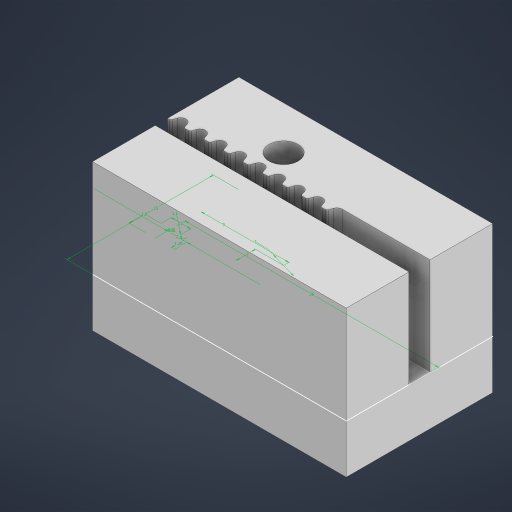
# Autodesk Inventor part: Y Axis Carriage
Saved by Autodesk Inventor 2024 (Build 280153000, 153)
## iProperties
Created: 2024-10-02
Part Number: Y Axis Carriage
Material: Generic
Document SubType Name: Modeling
Designer: jerem
Density: 1 g/cm^3
Appearance: Default
Author: jerem
Autodesk Inventor part; units mm, degrees
ref_plane "YZ Plane" through (0, 0, 0) normal (1, 0, 0) x (0, 1, 0)
ref_plane "XZ Plane" through (0, 0, 0) normal (0, 1, 0) x (-1, 0, 0)
ref_plane "XY Plane" through (0, 0, 0) normal (0, 0, 1) x (1, 0, 0)
sketch "Sketch1" plane through (0, 0, 0) normal (0, 1, 0) x (-1, 0, 0)
  line L0 (0, 0) -> (0, -1.075)
  line L1 (0, 0) -> (0, 1.075) construction
  line L2 (0, -1.075) -> (-26, -1.075) construction
  line L3 (0, 1.075) -> (-26, 1.075)
  line L4 (0, 1.075) -> (0, 7.5) construction
  line L5 (0, -1.075) -> (0, -7.5) construction
  line L6 (-26, -1.075) -> (-26, 1.075)
  line L7 (0, 1.075) -> (0, 7.5)
  line L8 (0, 7.5) -> (-26, 7.5)
  line L9 (-26, 7.5) -> (-26, 1.075)
  line L10 (0, -7.5) -> (-26, -7.5)
  line L11 (-26, -7.5) -> (-26, -1.075)
  line L12 (1, -0.525) -> (1, 1.075) construction
  arc A0 (-1.5221, -0.698) -> (-0.4779, -0.698) centre (-1, -0.525) ccw
  line L13 (0, -0.175) -> (-0.1602, -0.175)
  line L14 (-0.35, -0.3121) -> (-0.4779, -0.698)
  line L15 (-1, -0.525) -> (1, -0.525) construction
  line L16 (0, -0.525) -> (0, -0.175) construction
  arc A1 (-0.1602, -0.175) -> (-0.35, -0.3121) centre (-0.1602, -0.375) ccw
  line L17 (-1, -0.525) -> (-1, 0) construction
  line L18 (-1, -0.525) -> (-1, 0.025) construction
  line L19 (-2, -0.175) -> (-1.8398, -0.175)
  line L20 (-1.65, -0.3121) -> (-1.5221, -0.698)
  arc A2 (-1.65, -0.3121) -> (-1.8398, -0.175) centre (-1.8398, -0.375) ccw
  line L21 (-2, -0.175) -> (-2.1602, -0.175)
  arc A3 (-2.1602, -0.175) -> (-2.35, -0.3121) centre (-2.1602, -0.375) ccw
  line L22 (-2.35, -0.3121) -> (-2.4779, -0.698)
  arc A4 (-3.5221, -0.698) -> (-2.4779, -0.698) centre (-3, -0.525) ccw
  line L23 (-3.65, -0.3121) -> (-3.5221, -0.698)
  arc A5 (-3.65, -0.3121) -> (-3.8398, -0.175) centre (-3.8398, -0.375) ccw
  line L24 (-4, -0.175) -> (-3.8398, -0.175)
  line L25 (-4, -0.175) -> (-4.1602, -0.175)
  arc A6 (-4.1602, -0.175) -> (-4.35, -0.3121) centre (-4.1602, -0.375) ccw
  line L26 (-4.35, -0.3121) -> (-4.4779, -0.698)
  arc A7 (-5.5221, -0.698) -> (-4.4779, -0.698) centre (-5, -0.525) ccw
  line L27 (-5.65, -0.3121) -> (-5.5221, -0.698)
  arc A8 (-5.65, -0.3121) -> (-5.8398, -0.175) centre (-5.8398, -0.375) ccw
  line L28 (-6, -0.175) -> (-5.8398, -0.175)
  line L29 (-6, -0.175) -> (-6.1602, -0.175)
  arc A9 (-6.1602, -0.175) -> (-6.35, -0.3121) centre (-6.1602, -0.375) ccw
  line L30 (-6.35, -0.3121) -> (-6.4779, -0.698)
  arc A10 (-7.5221, -0.698) -> (-6.4779, -0.698) centre (-7, -0.525) ccw
  line L31 (-7.65, -0.3121) -> (-7.5221, -0.698)
  arc A11 (-7.65, -0.3121) -> (-7.8398, -0.175) centre (-7.8398, -0.375) ccw
  line L32 (-8, -0.175) -> (-7.8398, -0.175)
  line L33 (-8, -0.175) -> (-8.1602, -0.175)
  arc A12 (-8.1602, -0.175) -> (-8.35, -0.3121) centre (-8.1602, -0.375) ccw
  line L34 (-8.35, -0.3121) -> (-8.4779, -0.698)
  arc A13 (-9.5221, -0.698) -> (-8.4779, -0.698) centre (-9, -0.525) ccw
  line L35 (-9.65, -0.3121) -> (-9.5221, -0.698)
  arc A14 (-9.65, -0.3121) -> (-9.8398, -0.175) centre (-9.8398, -0.375) ccw
  line L36 (-10, -0.175) -> (-9.8398, -0.175)
  line L37 (-10, -0.175) -> (-10.1602, -0.175)
  arc A15 (-10.1602, -0.175) -> (-10.35, -0.3121) centre (-10.1602, -0.375) ccw
  line L38 (-10.35, -0.3121) -> (-10.4779, -0.698)
  arc A16 (-11.5221, -0.698) -> (-10.4779, -0.698) centre (-11, -0.525) ccw
  line L39 (-11.65, -0.3121) -> (-11.5221, -0.698)
  arc A17 (-11.65, -0.3121) -> (-11.8398, -0.175) centre (-11.8398, -0.375) ccw
  line L40 (-12, -0.175) -> (-11.8398, -0.175)
  line L41 (-12, -0.175) -> (-12.1602, -0.175)
  arc A18 (-12.1602, -0.175) -> (-12.35, -0.3121) centre (-12.1602, -0.375) ccw
  line L42 (-12.35, -0.3121) -> (-12.4779, -0.698)
  arc A19 (-13.5221, -0.698) -> (-12.4779, -0.698) centre (-13, -0.525) ccw
  line L43 (-13.65, -0.3121) -> (-13.5221, -0.698)
  arc A20 (-13.65, -0.3121) -> (-13.8398, -0.175) centre (-13.8398, -0.375) ccw
  line L44 (-14, -0.175) -> (-13.8398, -0.175)
  line L45 (-14, -0.175) -> (-14.1602, -0.175)
  arc A21 (-14.1602, -0.175) -> (-14.35, -0.3121) centre (-14.1602, -0.375) ccw
  line L46 (-14.35, -0.3121) -> (-14.4779, -0.698)
  arc A22 (-15.5221, -0.698) -> (-14.4779, -0.698) centre (-15, -0.525) ccw
  line L47 (-15.65, -0.3121) -> (-15.5221, -0.698)
  arc A23 (-15.65, -0.3121) -> (-15.8398, -0.175) centre (-15.8398, -0.375) ccw
  line L48 (-16, -0.175) -> (-15.8398, -0.175)
  line L49 (-16, -0.175) -> (-16, -1.075) construction
  circle A24 centre (-9, -3.075) radius 1.5
  line L50 (-16, -1.075) -> (-26, -1.075)
  line L51 (0, -1.075) -> (0, -7.5)
  line L52 (-9, -3.075) -> (-9, -1.075) construction
  arc A25 (-17, -1.075) -> (-16.4779, -0.698) centre (-17, -0.525) ccw
  line L53 (-16.35, -0.3121) -> (-16.4779, -0.698)
  arc A26 (-16.1602, -0.175) -> (-16.35, -0.3121) centre (-16.1602, -0.375) ccw
  line L54 (-16, -0.175) -> (-16.1602, -0.175)
  line L55 (0, 0) -> (0, 1.075)
  point P0 (0, -0.5375)
  point P1 (-0.3046, -0.175)
  point P2 (-2.3046, -0.175)
  point P3 (-4.3046, -0.175)
  point P4 (-6.3046, -0.175)
  point P5 (-8.3046, -0.175)
  point P6 (-10.3046, -0.175)
  point P7 (-12.3046, -0.175)
  point P8 (-14.3046, -0.175)
  point P9 (-17.5221, -0.698)
  dimension "d7" = 26
  dimension "d8" = 15
  dimension "d10" = 1.6
  dimension "d12" = 1.1
  dimension "d13" = 2
  dimension "d14" = 1.25
  dimension "d17" = 0.35
  dimension "d18" = 0.2
  dimension "d21" = 2
  dimension "d26" = 3
  dimension "d28" = 2
  dimension "d29" = 9
  constraints: 112 end point, 52 point on circle, 27 centre point, 23 point on line, 11 symmetric about line, 8 perpendicular, 7 vertical, 6 horizontal, 4 tangent, 3 collinear, 3 equal length, 2 midpoint, 136 other
  measures "d7" distance of L0.end L2.end
  measures "d8" distance of L4.end L5.end
  measures "d10" distance of L12.start L12.end
  measures "d12" diameter of A0
  measures "d13" distance of L15.start L12.start
  measures "d14" distance between parallel lines of L3 L13
  measures "d17" horizontal distance of L13.start L14.start
  measures "d18" distance of L13.end A1.centre
  measures "d21" distance of L13.start L21.start
  measures "d26" diameter of A24
  measures "d28" distance from line of L2 L52.start
  measures "d29" distance between parallel lines of L5 L52
extrude "Extrusion2" add sketch "Sketch1" along normal blind 10 contours L0 L51 L10 L11 L50 A25 L53 A26 L54 L48 A23 L47 A22 L46 A21 L45 L44 A20 L43 A19 L42 A18 L41 L40 A17 L39 A16 L38 A15 L37 L36 A14 L35 A13 L34 A12 L33 L32 A11 L31 A10 L30 A9 L29 L28 A8 L27 A7 L26 A6 L25 L24 A5 L23 A4 L22 A3 L21 L19 A2 L20 A0 L14 A1 L13 | L3 L9 L8 L7
extrude "Extrusion3" add sketch "Sketch1" against normal blind 5 contours L0 L13 A1 L14 A0 L20 A2 L19 L21 A3 L22 A4 L23 A5 L24 L25 A6 L26 A7 L27 A8 L28 L29 A9 L30 A10 L31 A11 L32 L33 A12 L34 A13 L35 A14 L36 L37 A15 L38 A16 L39 A17 L40 L41 A18 L42 A19 L43 A20 L44 L45 A21 L46 A22 L47 A23 L48 L54 A26 L53 A25 L50 L6 L3 L55 | L0 L51 L10 L11 L50 A25 L53 A26 L54 L48 A23 L47 A22 L46 A21 L45 L44 A20 L43 A19 L42 A18 L41 L40 A17 L39 A16 L38 A15 L37 L36 A14 L35 A13 L34 A12 L33 L32 A11 L31 A10 L30 A9 L29 L28 A8 L27 A7 L26 A6 L25 L24 A5 L23 A4 L22 A3 L21 L19 A2 L20 A0 L14 A1 L13 | L3 L9 L8 L7 | A24
body "Solid2"
